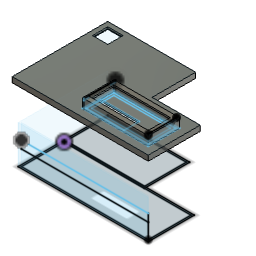
holder_lid_p1_p2 (Autodesk Fusion 360 design; units mm, degrees)
Autodesk Fusion 360 part; units mm, degrees
sketch "Sketch1" plane through (0, 0, 0) normal (0, 1, 0) x (1, 0, 0)
  line L0 (0, 0) -> (166, 0)
  line L1 (166, 0) -> (166, -56)
  line L2 (166, -56) -> (0, -56)
  line L3 (0, -56) -> (0, 0)
  line L4 (168, -58) -> (-2, -58)
  line L5 (-2, -58) -> (-2, 2)
  line L6 (-2, 2) -> (168, 2)
  line L7 (168, 2) -> (168, -58)
  line L8 (0, 2) -> (103, 2)
  line L9 (103, 2) -> (103, 57)
  line L10 (103, 57) -> (0, 57)
  line L11 (0, 57) -> (0, 2)
  line L12 (105, 0) -> (105, 59)
  line L13 (105, 59) -> (-2, 59)
  line L14 (-2, 59) -> (-2, 0)
  line L15 (-2, 0) -> (105, 0)
  line L16 (0, 2) -> (0, 0)
  dimension "d1" = 166
  dimension "d2" = 56
  dimension "d3" = -2
  dimension "d4" = 103
  dimension "d5" = 55
  dimension "d6" = 2
  constraint horizontal L0
  constraint vertical L1
  constraint horizontal L2
  constraint vertical L3
  constraint coincident L0.start L3.end
  constraint horizontal L8
  constraint vertical L9
  constraint horizontal L10
  constraint vertical L11
  constraint coincident L6 L8.start
  constraint perpendicular L0 L16
  measures "d1" distance of L0.start L0.end
  measures "d2" distance of L0.start L2.end
  measures "d4" distance of L8.start L8.end
  measures "d5" distance of L8.start L10.end
extrude "Extrude1" add sketch "Sketch1" along normal blind 50 contours L6 L9 L10 L11 L12 L13 L14 makes body 1
extrude "Extrude2" add sketch "Sketch1" along normal blind 10 contours L0 L6 L8 L12 L15 L16 | L5 L6 L14 L15 L16 bodies 1
extrude "Extrude3" add sketch "Sketch1" along normal blind 50 separate body contours L0 L1 L2 L3 L4 L5 L6 L7 L12 L15 makes body 2
extrude "Extrude4" add 1 faces at (-1.3333, 23.3333, -2) along direction (0, 0, 1) blind 2 on bodies 1 bodies 1 2
extrude "Extrude5" add sketch "Sketch1" against normal blind 2 separate body makes body 3
sketch "Sketch2" plane through (-2, 0, 0) normal (-1, 0, 0) x (0, 0, 1)
  line L0 (-59, 0) -> (58, 0)
  line L1 (58, 0) -> (58, 50)
  line L2 (58, 50) -> (-59, 50)
  line L3 (-59, 50) -> (-59, 0)
sketch "Sketch3" plane through (0, 0, 0) normal (1, 0, 0) x (0, 0, -1)
  line L0 (2, 0) -> (57, 0)
  line L1 (57, 0) -> (57, 50)
  line L2 (57, 50) -> (-56, 50)
  line L3 (-56, 50) -> (-56, 0)
  line L4 (-56, 0) -> (0, 0)
  line L5 (0, 0) -> (0, 10)
  line L6 (0, 10) -> (2, 10)
  line L7 (2, 10) -> (2, 0)
  line L8 (2, 0) -> (57, 0)
  line L9 (57, 0) -> (57, 20)
  line L10 (57, 20) -> (2, 20)
  line L11 (2, 20) -> (2, 0)
  dimension "d17" = 20
  constraint horizontal L8
  constraint vertical L9
  constraint horizontal L10
  constraint vertical L11
  constraint coincident L1 L9.end
  constraint coincident L0.start L7.end
  measures "d17" distance of L0.start L10.end
extrude "Extrude6" cut sketch "Sketch3" against normal blind 2 contours L0 L1 L7 L8 L9 L10 L11 bodies 1
extrude "Extrude7" add 1 faces at (103.6667, 23.3333, -2) along direction (0, 0, 1) blind 2 on bodies 1 bodies 1
sketch "Sketch4" plane through (0, 50, 0) normal (0, 1, 0) x (-1, 0, 0)
  line L0 (-105, -2) -> (-105, -59)
  line L1 (-105, -59) -> (2, -59)
  line L2 (2, -59) -> (2, 58)
  line L3 (2, 58) -> (-168, 58)
  line L4 (-168, 58) -> (-168, -2)
  line L5 (-168, -2) -> (-105, -2)
  line L6 (-103, -57) -> (-103, 0)
  line L7 (-103, 0) -> (-166, 0)
  line L8 (-166, 0) -> (-166, 56)
  line L9 (-166, 56) -> (0, 56)
  line L10 (0, 56) -> (0, -57)
  line L11 (0, -57) -> (-103, -57)
  line L12 (2, 58) -> (2, 8)
  line L13 (0, 8) -> (-168, 8)
  line L14 (2, 8) -> (0, 8)
  dimension "d22" = 50
  constraint coincident L2.end L3.start
  constraint perpendicular L3 L12
  constraint coincident L10 L13.start
  constraint coincident L4 L13.end
  constraint perpendicular L4 L13
  constraint perpendicular L10 L14
  measures "d22" distance of L2.end L12.end
sketch "Sketch5" plane through (0, 50, 0) normal (0, 1, 0) x (-1, 0, 0)
sketch "Sketch6" plane through (0, 0, 58) normal (0, 0, 1) x (1, 0, 0)
  line L0 (-2, 0) -> (168, 0)
  line L1 (168, 0) -> (168, 50)
  line L2 (168, 50) -> (-2, 50)
  line L3 (-2, 50) -> (-2, 0)
sketch "Sketch7" plane through (0, 0, 56) normal (0, 0, -1) x (-1, 0, 0)
  line L0 (-166, 0) -> (0, 0)
  line L1 (0, 0) -> (0, 50)
  line L2 (0, 50) -> (-166, 50)
  line L3 (-166, 50) -> (-166, 0)
  line L4 (-166, 0) -> (-166, 20)
  line L5 (-166, 20) -> (0, 20)
  line L6 (0, 20) -> (0, 30)
  line L7 (0, 30) -> (-166, 30)
  line L8 (-166, 30) -> (-166, 20)
  dimension "d24" = 20
  constraint coincident L0.start L3.end
  constraint perpendicular L0 L4
  constraint horizontal L5
  constraint vertical L6
  constraint horizontal L7
  constraint vertical L8
  constraint coincident L1 L6.end
  measures "d24" distance of L0.start L4.end
extrude "Extrude8" cut sketch "Sketch7" against normal blind 2 contours L1 L3 L5 L6 L7 L8 bodies 1
extrude "Extrude9" add 1 faces at (110.6667, 50, 57.3333) along direction (0, 1, 0) blind 50 on bodies 1 bodies 1
sketch "Sketch8" plane through (0, -2, 0) normal (0, -1, 0) x (1, 0, 0)
  line L0 (105, -59) -> (105, -2)
  line L1 (105, -2) -> (168, -2)
  line L2 (168, -2) -> (168, 58)
  line L3 (168, 58) -> (-2, 58)
  line L4 (-2, 58) -> (-2, -59)
  line L5 (-2, -59) -> (105, -59)
  circle A0 centre (0, 80) radius 15
  circle A1 centre (40, 80) radius 15
  circle A2 centre (80, 80) radius 15
  circle A3 centre (120, 80) radius 15
  circle A4 centre (160, 80) radius 15
  circle A5 centre (200, 80) radius 15
  circle A6 centre (-40, 80) radius 15
  circle A7 centre (-80, 80) radius 15
  circle A8 centre (-120, 80) radius 15
  circle A9 centre (-160, 80) radius 15
  circle A10 centre (240, 80) radius 15
  circle A11 centre (280, 80) radius 15
  circle A12 centre (320, 80) radius 15
  circle A13 centre (360, 80) radius 15
  circle A14 centre (-200, 80) radius 15
  circle A15 centre (400, 80) radius 15
  circle A16 centre (-240, 80) radius 15
  line L6 (-260, 60) -> (420, 60)
  line L7 (420, 60) -> (420, 100)
  line L8 (420, 100) -> (-260, 100)
  line L9 (-260, 100) -> (-260, 60)
  dimension "d29" = 30
  dimension "d30" = 30
  dimension "d31" = 30
  dimension "d32" = 30
  dimension "d33" = 30
  dimension "d34" = 30
  dimension "d35" = 30
  dimension "d36" = 30
  dimension "d37" = 30
  dimension "d38" = 30
  dimension "d39" = 30
  dimension "d40" = 30
  dimension "d41" = 30
  dimension "d42" = 30
  dimension "d43" = 30
  dimension "d44" = 30
  dimension "d45" = 30
  constraint horizontal L6
  constraint vertical L7
  constraint horizontal L8
  constraint vertical L9
  measures "d29" diameter of A0
  measures "d30" diameter of A1
  measures "d31" diameter of A2
  measures "d32" diameter of A3
  measures "d33" diameter of A4
  measures "d34" diameter of A5
  measures "d35" diameter of A6
  measures "d36" diameter of A7
  measures "d37" diameter of A8
  measures "d38" diameter of A9
  measures "d39" diameter of A10
  measures "d40" diameter of A11
  measures "d41" diameter of A12
  measures "d42" diameter of A13
  measures "d43" diameter of A14
  measures "d44" diameter of A15
  measures "d45" diameter of A16
sketch "Sketch9" plane through (0, 43, 0) normal (0, -1, 0) x (1, 0, 0)
  circle A0 centre (-120, 80) radius 15
  circle A1 centre (-40, 80) radius 15
  circle A2 centre (0, 80) radius 15
  circle A3 centre (120, 80) radius 15
  circle A4 centre (160, 80) radius 15
  circle A5 centre (-160, 80) radius 15
  circle A6 centre (80, 80) radius 15
  circle A7 centre (40, 80) radius 15
  circle A8 centre (240, 80) radius 15
  circle A9 centre (200, 80) radius 15
  circle A10 centre (-80, 80) radius 15
  circle A11 centre (-200, 80) radius 15
  circle A12 centre (360, 80) radius 15
  circle A13 centre (320, 80) radius 15
  circle A14 centre (-240, 80) radius 15
  circle A15 centre (280, 80) radius 15
  circle A16 centre (400, 80) radius 15
  line L0 (-260, 100) -> (-260, 60)
  line L1 (-260, 60) -> (420, 60)
  line L2 (420, 60) -> (420, 100)
  line L3 (420, 100) -> (-260, 100)
  line L4 (-260, 100) -> (420, 100)
  line L5 (420, 100) -> (420, 60)
  line L6 (420, 60) -> (-260, 60)
  line L7 (-260, 60) -> (-260, 100)
  line L8 (418, 62) -> (-258, 62)
  line L9 (-258, 62) -> (-258, 98)
  line L10 (-258, 98) -> (418, 98)
  line L11 (418, 98) -> (418, 62)
  dimension "d50" = 2
  constraint horizontal L4
  constraint vertical L5
  constraint horizontal L6
  constraint vertical L7
  constraint coincident L1.end L2.start
  constraint coincident L0.start L3.end
ref_plane "WorkPlane1" through (83, 101, -0.5) normal (0, 1, 0) x (0, 0, 1)
sketch "Sketch15" plane through (0, 101, 0) normal (0, 1, 0) x (1, 0, 0)
sketch "Sketch16" plane through (0, 100, 0) normal (0, 1, 0) x (-1, 0, 0)
  line L0 (-105, -2) -> (-105, -59)
  line L1 (-105, -59) -> (2, -59)
  line L2 (2, -59) -> (2, 58)
  line L3 (2, 58) -> (-168, 58)
  line L4 (-168, 58) -> (-168, -2)
  line L5 (-168, -2) -> (-105, -2)
  line L6 (-103, -57) -> (-103, 0)
  line L7 (-103, 0) -> (-166, 0)
  line L8 (-166, 0) -> (-166, 56)
  line L9 (-166, 56) -> (0, 56)
  line L10 (0, 56) -> (0, -57)
  line L11 (0, -57) -> (-103, -57)
  line L12 (2, -59) -> (-105, -59)
  line L13 (-105, -59) -> (-105, 0)
  line L14 (-105, 0) -> (2, 0)
  line L15 (2, 0) -> (2, -59)
  line L16 (-105, 0) -> (2, 0)
  line L17 (2, 0) -> (2, -2)
  line L18 (2, -2) -> (-105, -2)
  line L19 (-105, -2) -> (-105, 0)
  line L20 (2, 0) -> (-166, 0)
  line L21 (-166, 0) -> (-166, 56)
  line L22 (-166, 56) -> (2, 56)
  line L23 (2, 56) -> (2, 0)
  line L24 (2, -2) -> (-168, -2)
  line L25 (-168, -2) -> (-168, 58)
  line L26 (-168, 58) -> (2, 58)
  line L27 (2, 58) -> (2, -2)
  line L28 (4, 0) -> (4, -61)
  line L29 (4, -61) -> (-107, -61)
  line L30 (-107, -61) -> (-107, 0)
  line L31 (4, -4) -> (-170, -4)
  line L32 (-170, -4) -> (-170, 60)
  line L33 (-170, 60) -> (4, 60)
  line L34 (4, 60) -> (4, -4)
  line L35 (6, 0) -> (6, -63)
  line L36 (6, -63) -> (-109, -63)
  line L37 (-109, -63) -> (-109, 0)
  line L38 (6, -6) -> (-172, -6)
  line L39 (-172, -6) -> (-172, 62)
  line L40 (-172, 62) -> (6, 62)
  line L41 (6, 62) -> (6, -6)
  dimension "d60" = 2
  dimension "d61" = -2
  dimension "d62" = -2
  dimension "d65" = -4
  dimension "d66" = -4
  constraint horizontal L12
  constraint vertical L13
  constraint horizontal L14
  constraint vertical L15
  constraint coincident L7 L13.end
  constraint coincident L1.end L2.start
  constraint horizontal L16
  constraint vertical L17
  constraint horizontal L18
  constraint vertical L19
  constraint horizontal L20
  constraint vertical L21
  constraint horizontal L22
  constraint vertical L23
  constraint coincident L8.end L9.start
  constraint horizontal L24
  constraint vertical L25
  constraint horizontal L26
  constraint vertical L27
  constraint coincident L3.end L4.start
  measures "d60" distance of L13.end L0.start
sketch "Sketch18" plane through (0, 100, 0) normal (0, 1, 0) x (-1, 0, 0)
extrude "Extrude16" add sketch "Sketch16" along normal blind 2 separate body makes body 4
extrude "Extrude17" add sketch "Sketch16" against normal blind 5 contours L30 L31 L37 L38 | L28 L29 L30 L35 L36 L37 L38 | L28 L31 L32 L33 L34 L35 L37 L38 L39 L40 L41 bodies 4
sketch "Sketch19" plane through (0, 100, 0) normal (0, 1, 0) x (-1, 0, 0)
  line L0 (-0.0472, -57.0294) -> (-20.0472, -57.0294)
  line L1 (-20.0472, -57.0294) -> (-20.0472, -37.0294)
  line L2 (-20.0472, -37.0294) -> (-0.0472, -37.0294)
  line L3 (-0.0472, -37.0294) -> (-0.0472, -57.0294)
  dimension "d71" = 20
  dimension "d72" = 20
  constraint horizontal L0
  constraint vertical L1
  constraint horizontal L2
  constraint vertical L3
  measures "d71" distance of L0.start L0.end
  measures "d72" distance of L0.start L2.end
extrude "Extrude18" cut sketch "Sketch19" along normal blind 2 bodies 4
sketch "Sketch20" plane through (0, 102, 0) normal (0, 1, 0) x (-1, 0, 0)
  line L0 (-0.0472, -37.0294) -> (-0.0472, -57.0294)
  line L1 (-0.0472, -57.0294) -> (-20.0472, -57.0294)
  line L2 (-20.0472, -57.0294) -> (-20.0472, -37.0294)
  line L3 (-20.0472, -37.0294) -> (-0.0472, -37.0294)
  line L4 (6, 62) -> (-172, 62)
  line L5 (-172, 62) -> (-172, -6)
  line L6 (-172, -6) -> (-109, -6)
  line L7 (-109, -6) -> (-109, -63)
  line L8 (-109, -63) -> (6, -63)
  line L9 (6, -63) -> (6, 62)
  line L10 (-160, 50) -> (-78, 50)
  line L11 (-78, 50) -> (-78, 13)
  line L12 (-78, 13) -> (-160, 13)
  line L13 (-160, 13) -> (-160, 50)
  line L14 (-82, 17) -> (-156, 17)
  line L15 (-156, 17) -> (-156, 46)
  line L16 (-156, 46) -> (-82, 46)
  line L17 (-82, 46) -> (-82, 17)
  line L18 (-162, 52) -> (-76, 52)
  line L19 (-76, 52) -> (-76, 11)
  line L20 (-76, 11) -> (-162, 11)
  line L21 (-162, 11) -> (-162, 52)
  line L22 (-78, 50) -> (-128, 50)
  line L23 (-128, 50) -> (-128, 30)
  line L24 (-128, 30) -> (-78, 30)
  line L25 (-78, 30) -> (-78, 50)
  line L26 (-79, 14) -> (-159, 14)
  line L27 (-159, 14) -> (-159, 49)
  line L28 (-159, 49) -> (-79, 49)
  line L29 (-79, 49) -> (-79, 14)
  dimension "d75" = 82
  dimension "d76" = 37
  dimension "d77" = 4
  dimension "d78" = -2
  dimension "d92" = 50
  dimension "d93" = 20
  dimension "d94" = 1
  constraint horizontal L10
  constraint vertical L11
  constraint horizontal L12
  constraint vertical L13
  constraint horizontal L22
  constraint vertical L23
  constraint horizontal L24
  constraint vertical L25
  measures "d75" distance of L10.start L10.end
  measures "d76" distance of L10.start L12.end
  measures "d92" distance of L10.end L22.end
  measures "d93" distance of L10.end L24.end
extrude "Extrude19" add sketch "Sketch20" along normal blind 8 contours L18 L19 L20 L21 bodies 4
extrude "Extrude20" add 1 faces at (105.3333, 110, 11.6667) along direction (0, 1, 0) blind 4 on bodies 4 bodies 4
sketch "Sketch21" plane through (160, 0, 0) normal (-1, 0, 0) x (0, 0, 1)
  line L0 (13, 102) -> (50, 102)
  line L1 (50, 102) -> (50, 114)
  line L2 (50, 114) -> (13, 114)
  line L3 (13, 114) -> (13, 102)
  line L4 (13, 114) -> (50, 114)
  line L5 (50, 114) -> (50, 112)
  line L6 (50, 112) -> (13, 112)
  line L7 (13, 112) -> (13, 114)
  line L8 (13, 114) -> (17, 114)
  line L9 (17, 114) -> (17, 112)
  line L10 (17, 112) -> (13, 112)
  line L11 (13, 112) -> (13, 114)
  line L12 (50, 114) -> (46, 114)
  line L13 (46, 114) -> (46, 112)
  line L14 (46, 112) -> (50, 112)
  line L15 (50, 112) -> (50, 114)
  dimension "d83" = 2
  dimension "d84" = 4
  dimension "d85" = 4
  constraint horizontal L4
  constraint vertical L5
  constraint horizontal L6
  constraint vertical L7
  constraint coincident L1 L5.end
  constraint coincident L2.end L3.start
  constraint horizontal L8
  constraint vertical L9
  constraint horizontal L10
  constraint vertical L11
  constraint horizontal L12
  constraint vertical L13
  constraint horizontal L14
  constraint vertical L15
  constraint coincident L1.end L2.start
  measures "d83" distance of L2.end L6.end
  measures "d84" distance of L2.end L8.end
  measures "d85" distance of L1.end L12.end
extrude "Extrude21" add sketch "Sketch21" along normal blind 4 contours L2 L4 L6 L9 L13 bodies 4
extrude "Extrude22" add sketch "Sketch21" along normal blind 82 contours L2 L3 L4 L6 L7 L8 L9 L10 L11 | L1 L2 L4 L5 L6 L12 L13 L14 L15 bodies 4
extrude "Extrude23" cut 1 faces at (76, 106, 38.3333) along direction (1, 0, 0) blind 2 on bodies 4 bodies 4
extrude "Extrude24" cut sketch "Sketch20" against normal blind 2 contours L16 L17 L23 L24 L28 L29 | L16 L17 L23 L24 bodies 4
sketch "Sketch22" plane through (78, 0, 0) normal (-1, 0, 0) x (0, 0, 1)
  line L0 (17, 112) -> (17, 114)
  line L1 (17, 114) -> (11, 114)
  line L2 (11, 114) -> (11, 102)
  line L3 (11, 102) -> (13, 102)
  line L4 (13, 102) -> (13, 112)
  line L5 (13, 112) -> (17, 112)
  line L6 (11, 114) -> (52, 114)
  line L7 (52, 114) -> (52, 102)
  line L8 (52, 102) -> (11, 102)
  line L9 (11, 102) -> (11, 114)
  line L10 (11, 114) -> (52, 114)
  line L11 (52, 114) -> (52, 112)
  line L12 (52, 112) -> (11, 112)
  line L13 (11, 112) -> (11, 114)
  line L14 (11, 114) -> (17, 114)
  line L15 (17, 114) -> (17, 112)
  line L16 (17, 112) -> (11, 112)
  line L17 (11, 112) -> (11, 114)
  line L18 (52, 114) -> (46, 114)
  line L19 (46, 114) -> (46, 112)
  line L20 (46, 112) -> (52, 112)
  line L21 (52, 112) -> (52, 114)
  dimension "d97" = 41
  dimension "d98" = 12
  dimension "d99" = 2
  dimension "d100" = 6
  dimension "d101" = 6
  constraint horizontal L6
  constraint vertical L7
  constraint horizontal L8
  constraint vertical L9
  constraint coincident L1.end L2.start
  constraint horizontal L10
  constraint vertical L11
  constraint horizontal L12
  constraint vertical L13
  constraint horizontal L14
  constraint vertical L15
  constraint horizontal L16
  constraint vertical L17
  constraint horizontal L18
  constraint vertical L19
  constraint horizontal L20
  constraint vertical L21
  measures "d97" distance of L1.end L6.end
  measures "d98" distance of L1.end L2.end
  measures "d99" distance of L1.end L12.end
  measures "d100" distance of L1.end L0.end
  measures "d101" distance of L6.end L18.end
sketch "Sketch23" plane through (78, 0, 0) normal (-1, 0, 0) x (0, 0, 1)
  line L0 (46, 114) -> (46, 112)
  line L1 (46, 112) -> (50, 112)
  line L2 (50, 112) -> (50, 102)
  line L3 (50, 102) -> (52, 102)
  line L4 (52, 102) -> (52, 114)
  line L5 (52, 114) -> (46, 114)
extrude "Extrude25" add sketch "Sketch22" sketch "Sketch23" along normal blind 2 separate body of sketch 2 makes body 5
extrude "Extrude26" add sketch "Sketch22" against normal blind 4 contours L0 L6 L10 L12 L15 L19 bodies 5
extrude "Extrude15" [rolled back] along distance 2 taper angle 0
sketch "Sketch17" plane through (0, 100, 0) normal (0, 1, 0) x (-1, 0, 0)
hidden bodies 1 3
